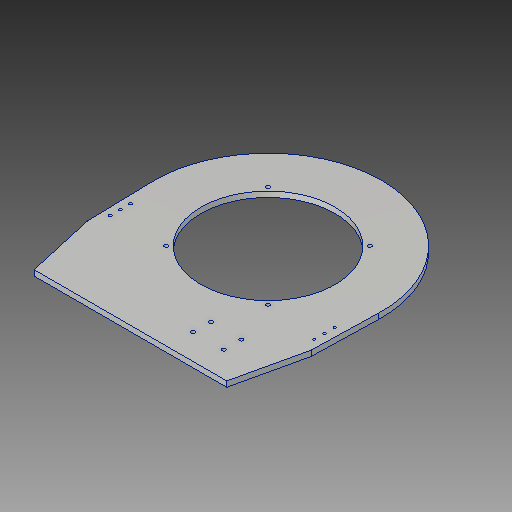
# Autodesk Inventor part: Turret Base Plate
Saved by Autodesk Inventor 2019.4 (Build 234330000, 330)
## iProperties
Created: 2020-01-06
Part Number: Turret Base Plate
Material: Aluminum 6061
Document SubType Name: Modeling
Designer: admin
Density: 2.7 g/cm^3
Appearance: Aluminum - Flat
Mass: 1633.61 g
Surface Area: 1675.58 cm^2
Volume: 605.039 cm^3
Author: admin
Autodesk Inventor part; units mm, degrees
ref_plane "YZ Plane" through (0, 0, 0) normal (1, 0, 0) x (0, 1, 0)
ref_plane "XZ Plane" through (0, 0, 0) normal (0, 1, 0) x (-1, 0, 0)
ref_plane "XY Plane" through (0, 0, 0) normal (0, 0, 1) x (1, 0, 0)
sketch "Sketch1" plane through (0, 0, 0) normal (0, 1, 0) x (-1, 0, 0)
  circle A0 centre (0, 0) radius 97.5
  arc A1 (164.9474, 4.1671) -> (-164.9474, 4.1671) centre (0, 0) ccw construction
  line L0 (-164.9474, 4.1671) -> (-160, 200)
  line L1 (-160, 200) -> (160, 200)
  line L2 (160, 200) -> (164.9474, 4.1671)
  line L3 (0, 200) -> (0, 0) construction
  arc A2 (-164.9474, 4.1671) -> (164.9474, 4.1671) centre (0, 0) ccw
  line L4 (-74, 74) -> (74, 74) construction
  line L5 (74, 74) -> (74, -74) construction
  line L6 (74, -74) -> (-74, -74) construction
  line L7 (-74, -74) -> (-74, 74) construction
  line L8 (-74, 74) -> (74, -74) construction
  line L9 (74, 74) -> (-74, -74) construction
  circle A3 centre (74, -74) radius 2.75
  circle A4 centre (-74, -74) radius 2.75
  circle A5 centre (-74, 74) radius 2.75
  circle A6 centre (74, 74) radius 2.75
  dimension "d0" = 195
  dimension "d1" = 330
  dimension "d2" = 200
  dimension "d3" = 320
  dimension "d6" = 148
  dimension "d7" = 5.5
  dimension "d8" = 5.5
  dimension "d9" = 5.5
  dimension "d10" = 5.5
  constraints: 20 end point, 7 centre point, 6 coincident, 4 point on circle, 3 midpoint, 3 perpendicular, 2 horizontal, 2 parallel, 2 tangent
  measures "d0" diameter of A0
  measures "d1" diameter of A1
  measures "d2" distance from line of L1 point (0, 0)
  measures "d3" distance of L0.end L1.end
  measures "d6" distance of L4.end L5.end
  measures "d7" diameter of A3
  measures "d8" diameter of A4
  measures "d9" diameter of A5
  measures "d10" diameter of A6
extrude "Extrusion1" add sketch "Sketch1" along normal blind 8
chamfer "Chamfer1" distance 100 distance2 20 1 edges at (-160, 4, 200) measured on face at (-160.0126, 4, 199.5002)
chamfer "Chamfer2" distance 20 distance2 100 1 edges at (160, 4, 200) measured on face at (159.5, 4, 200)
sketch "Sketch3" plane through (0, 0, 0) normal (0, -1, 0) x (1, 0, 0)
  circle A0 centre (54.0478, 137.3024) radius 2.0193 construction
  circle A1 centre (54.0478, 162.7024) radius 2.0193 construction
  circle A2 centre (98.4978, 162.7024) radius 2.0193 construction
  circle A3 centre (98.4978, 137.3024) radius 2.0193 construction
  circle A4 centre (151.3, 84.3853) radius 1.75 projected
  circle A5 centre (151.3, 69.3853) radius 1.75 projected
  line L0 (162.5255, 100.0319) -> (140, 200) projected
  line L1 (162.5255, 100.0319) -> (164.9474, 4.1671) projected
  arc A6 (-164.9474, 4.1671) -> (164.9474, 4.1671) centre (0, 0) ccw projected
  line L2 (-164.9474, 4.1671) -> (-162.5255, 100.0319) projected
  line L3 (-140, 200) -> (-162.5255, 100.0319) projected
  line L4 (-140, 200) -> (140, 200) projected
  circle A7 centre (0, 0) radius 97.5 projected
  circle A8 centre (-74, 74) radius 2.75 projected
  circle A9 centre (74, 74) radius 2.75 projected
  circle A10 centre (74, -74) radius 2.75 projected
  circle A11 centre (-74, -74) radius 2.75 projected
  circle A12 centre (151.3, 54.3853) radius 1.75 projected
  circle A13 centre (-152.8, 76.8815) radius 2.2 projected
  circle A14 centre (-152.8, 61.8815) radius 2.2 projected
  circle A15 centre (-152.8, 46.8815) radius 2.2 projected
  circle A16 centre (54.0478, 162.7024) radius 2.75
  circle A17 centre (98.4978, 162.7024) radius 2.75
  circle A18 centre (98.4978, 137.3024) radius 2.75
  circle A19 centre (54.0478, 137.3024) radius 2.75
  point P0 (0, 0)
  dimension "d19" = 5.5
  dimension "d20" = 5.5
  dimension "d21" = 5.5
  dimension "d22" = 5.5
  constraints: 4 centre point, 4 coincident
  measures "d19" diameter of A16
  measures "d20" diameter of A17
  measures "d21" diameter of A18
  measures "d22" diameter of A19
extrude "Extrusion3" cut sketch "Sketch3" against normal through all contours A4 | A5 | A12 | A13 | A14 | A15 | A16 | A17 | A18 | A19
chamfer "Chamfer3" distance 3 angle 45 14 edges at (-155, 0, 76.8815) (-155, 0, 61.8815) (-155, 0, 46.8815) (149.55, 0, 84.3853) (149.55, 0, 69.3853) (149.55, 0, 54.3853) (51.2978, 0, 137.3024) (95.7478, 0, 137.3024) (95.7478, 0, 162.7024) (51.2978, 0, 162.7024) (-71.25, 0, 74) (76.75, 0, 74) (76.75, 0, -74) (-71.25, 0, -74)
body "Solid1"
